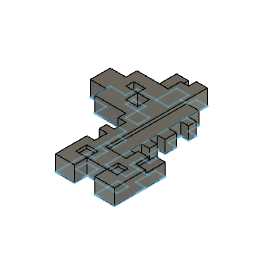
Giraffe-keychain (Autodesk Fusion 360 design; units mm, degrees)
Autodesk Fusion 360 part; units mm, degrees
sketch "giraffe" plane through (0, 0, 0) normal (0, 0, 1) x (1, 0, 0)
  line L0 (-42.5977, 27.0275) -> (-55, 27.0275)
  line L1 (-55, 27.0275) -> (-55, 20)
  line L2 (-55, 20) -> (-65, 20)
  line L3 (-65, 20) -> (-65, 7.3444)
  line L4 (-65, 7.3444) -> (-55, 7.3444)
  line L5 (-55, 7.3444) -> (-55, 0)
  line L6 (-55, 0) -> (-35, 0)
  line L7 (-35, 0) -> (-35, -45)
  line L8 (-35, -45) -> (-22.9146, -45)
  line L9 (-22.9146, -45) -> (-22.9146, -37.0159)
  line L10 (-9.9884, -37.0159) -> (-9.9884, -45)
  line L11 (-9.9884, -45) -> (2.644, -45)
  line L12 (2.644, -45) -> (2.644, -25)
  line L13 (2.644, -25) -> (-3.6722, -25)
  line L14 (-3.6722, -25) -> (-3.6722, -17.0391)
  line L15 (-3.6722, -17.0391) -> (-9.9884, -17.0391)
  line L16 (-9.9884, -17.0391) -> (-9.9884, -25)
  line L17 (-22.9146, -25) -> (-22.9146, 40)
  line L18 (-22.9146, 40) -> (-30, 40)
  line L19 (-30, 40) -> (-30, 35)
  line L20 (-30, 35) -> (-35, 35)
  line L21 (-35, 35) -> (-35, 27.0275)
  line L22 (-35, 27.0275) -> (-42.5977, 27.0275)
  line L23 (-42.5977, 27.0275) -> (-42.5977, 40)
  line L24 (-42.5977, 40) -> (-35, 40)
  line L25 (-35, 40) -> (-35, 35)
  line L26 (-22.9146, 26.7337) -> (-15, 26.7337)
  line L27 (-15, 26.7337) -> (-15, 20)
  line L28 (-15, 20) -> (-10, 20)
  line L29 (-10, 20) -> (-10, 15)
  line L30 (-10, 15) -> (-15, 15)
  line L31 (-15, 15) -> (-15, 7.3444)
  line L32 (-15, 7.3444) -> (-10, 7.3444)
  line L33 (-10, 7.3444) -> (-10, 0)
  line L34 (-10, 0) -> (-15, 0)
  line L35 (-15, 0) -> (-15, -5)
  line L36 (-15, -5) -> (-10, -5)
  line L37 (-10, -5) -> (-10, -10)
  line L38 (-10, -10) -> (-15, -10)
  line L39 (-15, -10) -> (-15, -15)
  line L40 (-15, -15) -> (-15, -17.0391)
  line L41 (-15, -17.0391) -> (-9.9884, -17.0391)
  line L42 (-3.6722, -17.0391) -> (-3.6722, -12.5)
  line L43 (-3.6722, -12.5) -> (0, -12.5)
  line L44 (0, -12.5) -> (2.644, -12.5)
  line L45 (2.644, -12.5) -> (2.644, -25)
  line L46 (-35, -5) -> (-30, -5)
  line L47 (-30, -5) -> (-30, -12.5)
  line L48 (-30, -12.5) -> (-35, -12.5)
  line L49 (-30, -30) -> (-30, -37.0159)
  line L50 (-30, -37.0159) -> (-22.9146, -37.0159)
  line L51 (-22.9146, -37.0159) -> (-22.9146, -30)
  line L52 (-22.9146, -30) -> (-30, -30)
  line L53 (-9.9884, -37.0159) -> (-9.9884, -30)
  line L54 (-9.9884, -37.0159) -> (-3.6722, -37.0159)
  line L55 (-3.6722, -37.0159) -> (-3.6722, -30)
  line L56 (-3.6722, -30) -> (-9.9884, -30)
  line L57 (-42.5977, 7.5) -> (-35, 7.5)
  line L58 (-35, 7.5) -> (-35, 15)
  line L59 (-35, 15) -> (-42.5977, 15)
  line L60 (-42.5977, 15) -> (-42.5977, 7.5)
  line L61 (-42.5977, 15) -> (-42.5977, 20)
  line L62 (-42.5977, 20) -> (-50, 20)
  line L63 (-50, 20) -> (-50, 15)
  line L64 (-50, 15) -> (-42.5977, 15)
  line L65 (-35, -25) -> (-30, -25)
  line L66 (-30, -25) -> (-30, -17.0391)
  line L67 (-30, -17.0391) -> (-35, -17.0391)
  line L68 (-22.9146, -25) -> (-9.9884, -25)
  line L69 (-22.9146, -37.0159) -> (-9.9884, -37.0159)
  constraint horizontal L0
  constraint perpendicular L0 L1
  constraint perpendicular L1 L2
  constraint perpendicular L2 L3
  constraint perpendicular L1 L4
  constraint perpendicular L4 L5
  constraint perpendicular L5 L6
  constraint perpendicular L6 L7
  constraint perpendicular L7 L8
  constraint perpendicular L8 L9
  constraint perpendicular L8 L10
  constraint perpendicular L10 L11
  constraint perpendicular L11 L12
  constraint perpendicular L12 L13
  constraint perpendicular L13 L14
  constraint perpendicular L12 L15
  constraint perpendicular L15 L16
  constraint perpendicular L15 L17
  constraint perpendicular L17 L18
  constraint perpendicular L18 L19
  constraint perpendicular L17 L20
  constraint perpendicular L20 L21
  constraint perpendicular L21 L22
  constraint perpendicular L22 L23
  constraint perpendicular L23 L24
  constraint perpendicular L20 L25
  constraint coincident L17 L26.start
  constraint perpendicular L17 L26
  constraint perpendicular L26 L27
  constraint perpendicular L27 L28
  constraint perpendicular L28 L29
  constraint perpendicular L29 L30
  constraint perpendicular L30 L31
  constraint perpendicular L31 L32
  constraint perpendicular L32 L33
  constraint perpendicular L33 L34
  constraint perpendicular L34 L35
  constraint perpendicular L35 L36
  constraint perpendicular L36 L37
  constraint perpendicular L37 L38
  constraint perpendicular L38 L39
  constraint perpendicular L38 L40
  constraint perpendicular L16 L41
  constraint perpendicular L15 L42
  constraint perpendicular L14 L43
  constraint perpendicular L42 L44
  constraint perpendicular L13 L45
  constraint coincident L7 L46.start
  constraint perpendicular L7 L46
  constraint perpendicular L46 L47
  constraint coincident L7 L48.end
  constraint perpendicular L7 L48
  constraint parallel L9 L49
  constraint perpendicular L9 L50
  constraint perpendicular L50 L51
  constraint perpendicular L49 L52
  constraint parallel L10 L53
  constraint perpendicular L10 L54
  constraint perpendicular L54 L55
  constraint perpendicular L53 L56
  constraint perpendicular L7 L57
  constraint perpendicular L57 L58
  constraint perpendicular L21 L59
  constraint perpendicular L57 L60
  constraint perpendicular L59 L61
  constraint perpendicular L61 L62
  constraint perpendicular L62 L63
  constraint perpendicular L60 L64
  constraint coincident L7 L65.start
  constraint perpendicular L7 L65
  constraint perpendicular L65 L66
  constraint coincident L7 L67.end
  constraint perpendicular L7 L67
  constraint perpendicular L16 L68
  constraint perpendicular L53 L69
extrude "Extrude1" add sketch "giraffe" along normal blind 10 contours L0 L1 L2 L3 L4 L5 L6 L7 L8 L9 L10 L11 L12 L13 L14 L15 L16 L17 L18 L19 L20 L21 L22 L46 L47 L48 L65 L66 L67 L68 L69 makes body 1
extrude "Extrude2" add sketch "giraffe" along normal blind 8 separate body contours L49 L50 L51 L52 | L53 L54 L55 L56 | L21 L22 L23 L24 L25 | L16 L17 L26 L27 L28 L29 L30 L31 L32 L33 L34 L35 L36 L37 L38 L39 L40 L41 L68 | L13 L14 L42 L43 L44 L45 makes body 2 at (-42.5977, 31.3517, 5.3333) makes body 3 at (-20.2764, 0.5779, 0) makes body 4 at (-27.6382, -37.0159, 2.6667) makes body 5 at (-3.6722, -20.8333, 5.3333) makes body 6 at (-9.9884, -34.6773, 2.6667)
combine "Combine1" operation add target body 5 tool bodies 2 3 1 6 4
named bodies: "Giraffe"
